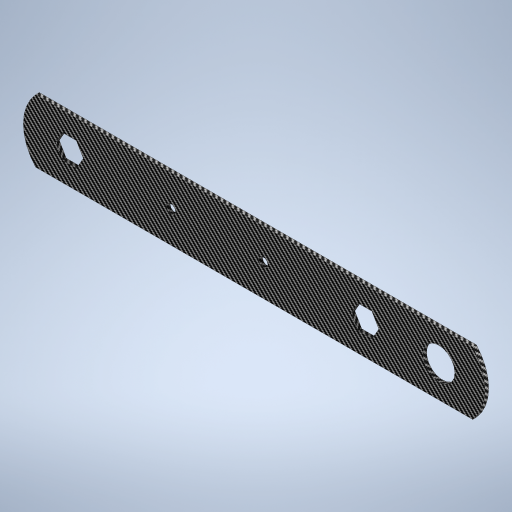
# Autodesk Inventor part: new arm plate
Saved by Autodesk Inventor 2023 (Build 270158000, 158)
## iProperties
Created: 2022-01-24
Part Number: new arm plate
Material: CFRP
Document SubType Name: Modeling
Designer: pauly
Density: 1.43 g/cm^3
Appearance: Carbon Fiber
Mass: 1188.25 g
Surface Area: 882.063 cm^2
Volume: 440.093 cm^3
Author: pauly
Autodesk Inventor part; units mm, degrees
ref_plane "YZ Plane" through (0, 0, 0) normal (1, 0, 0) x (0, 1, 0)
ref_plane "XZ Plane" through (0, 0, 0) normal (0, 1, 0) x (-1, 0, 0)
sketch "Sketch1" plane through (0, 0, 0) normal (0, 0, 1) x (1, 0, 0)
  line L0 (508.0015, 71.1714) -> (254.0015, 71.1714)
  circle A0 centre (508.0015, 39.4214) radius 10.9982
  arc A1 (254.0015, 71.1714) -> (254.0015, 7.6714) centre (254.0015, 39.4214) ccw
  arc A2 (508.0015, 7.6714) -> (508.0015, 71.1714) centre (508.0015, 39.4214) ccw
  line L1 (452.439, 47.6641) -> (461.964, 47.6641)
  line L2 (461.964, 47.6641) -> (466.7265, 39.4152)
  line L3 (461.964, 31.1664) -> (452.439, 31.1664)
  line L4 (452.439, 31.1664) -> (447.6765, 39.4152)
  line L5 (447.6765, 39.4152) -> (452.439, 47.6641)
  line L6 (466.7265, 39.4152) -> (461.964, 31.1664)
  line L7 (254.0015, 7.6714) -> (508.0015, 7.6714)
  line L8 (249.239, 47.6641) -> (258.764, 47.6641)
  line L9 (258.764, 47.6641) -> (263.5265, 39.4152)
  line L10 (263.5265, 39.4152) -> (258.764, 31.1664)
  line L11 (249.239, 47.6641) -> (244.4765, 39.4152)
  line L12 (244.4765, 39.4152) -> (249.239, 31.1664)
  line L13 (249.239, 31.1664) -> (258.764, 31.1664)
  circle A3 centre (323.8515, 39.4214) radius 3.175
  circle A4 centre (387.3515, 39.4214) radius 3.175
  point P0 (254.0015, 39.4214)
  point P1 (457.2015, 31.1664)
  point P2 (457.3274, 39.4214)
  dimension "d15" = 89.0524
  dimension "d18" = 44.45
  dimension "d36" = 56.5658
  dimension "d69" = 126.3396
  dimension "d72" = 25.4
  dimension "d3" = 21.9964
  dimension "d158" = 9.525
  dimension "d159" = 9.525
  dimension "d160" = 9.525
  dimension "d161" = 9.525
  dimension "d162" = 9.525
  dimension "d164" = 120
  dimension "d165" = 120
  dimension "d166" = 120
  dimension "d167" = 120
  dimension "d172" = 254
  dimension "d173" = 9.525
  dimension "d174" = 9.525
  dimension "d177" = 120
  dimension "d178" = 9.525
  dimension "d179" = 120
  dimension "d181" = 8.255
  dimension "d182" = 9.525
  dimension "d183" = 31.75
  dimension "d184" = 6.35
  dimension "d185" = 6.35
  dimension "d186" = 50.8
  dimension "d187" = 69.85
  dimension "d188" = 63.5
  dimension "d189" = 69.85
  dimension "d191" = 31.75
  dimension "d192" = 31.75
  dimension "d193" = 120
  dimension "d194" = 120
  dimension "d195" = 31.75
  dimension "d196" = 31.75
  dimension "d197" = 8.255
  dimension "d198" = 31.75
  constraints: 28 end point, 5 centre point, 5 horizontal, 4 point on circle, 4 tangent, 1 coincident, 1 midpoint
  measures "d3" diameter of A0
  measures "d158" distance of L1.start L1.end
  measures "d159" distance of L1.end L2.end
  measures "d160" distance of L3.start L3.end
  measures "d161" distance of L3.end L4.end
  measures "d162" distance of L4.end L1.start
  measures "d164" angle of L2 L1
  measures "d165" angle of L1 L5
  measures "d166" angle of L4 L5
  measures "d167" angle of L3 L4
  measures "d172" distance of L7.start L7.end
  measures "d173" distance of L8.start L8.end
  measures "d174" distance of L8.end L9.end
  measures "d177" angle of L9 L8
  measures "d178" distance of L9.end L10.end
  measures "d179" angle of L10 L9
  measures "d181" distance from line of L13 point (254.002, 39.421)
  measures "d182" distance of point (254.002, 39.421) L11.end
  measures "d183" distance of L0.end point (254.002, 39.421)
  measures "d184" diameter of A3
  measures "d185" diameter of A4
  measures "d186" horizontal distance of A0.centre point (457.202, 31.166)
  measures "d187" distance of A3.centre point (254.002, 39.421)
  measures "d188" distance of A4.centre A3.centre
  measures "d189" horizontal distance of point (457.202, 31.166) A4.centre
  measures "d191" radius of A2
  measures "d192" radius of A1
  measures "d193" angle of L12 L13
  measures "d194" angle of L11 L12
  measures "d195" distance from line of L7 A3.centre
  measures "d196" distance from line of L7 A4.centre
  measures "d197" distance from line of point (457.327, 39.421) L3
  measures "d198" distance from line of point (457.327, 39.421) L7
extrude "Extrusion10" add sketch "Sketch1" along normal blind 2.54
ref_plane "Work Plane1" through (0, 0, 1.27) normal (0, 0, 1) x (1, 0, 0)
sketch "Sketch2" plane through (0, 0, 1.27) normal (0, 0, 1) x (1, 0, 0)
  line L0 (193.0886, 111.8114) -> (574.0886, 111.8114)
  line L1 (574.0886, 111.8114) -> (574.0886, 61.0114)
  line L2 (574.0886, 61.0114) -> (193.0886, 61.0114)
  line L3 (193.0886, 61.0114) -> (193.0886, 111.8114)
  line L4 (194.851, 17.8314) -> (575.851, 17.8314)
  line L5 (575.851, 17.8314) -> (575.851, -32.9686)
  line L6 (575.851, -32.9686) -> (194.851, -32.9686)
  line L7 (194.851, -32.9686) -> (194.851, 17.8314)
  line L8 (508.0015, 71.1714) -> (254.0015, 71.1714) projected
  line L9 (254.0015, 7.6714) -> (508.0015, 7.6714) projected
  point P0 (0, 0)
  dimension "d199" = 381
  dimension "d200" = 50.8
  dimension "d201" = 381
  dimension "d202" = 50.8
  dimension "d203" = 53.34
  dimension "d204" = 53.34
  constraints: 16 end point, 4 parallel, 2 horizontal, 2 perpendicular
  measures "d199" distance of L0.start L0.end
  measures "d200" distance of L2.end L0.start
  measures "d201" distance of L5.end L6.end
  measures "d202" distance of L4.end L5.end
  measures "d203" distance between parallel lines of L8 L4
  measures "d204" distance between parallel lines of L2 L9
extrude "Extrusion11" cut sketch "Sketch2" along normal mid plane 25.4
body "Solid3"
